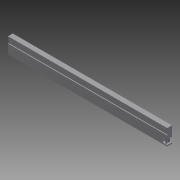
# Autodesk Inventor part: Bar
Saved by Autodesk Inventor 2012 (Build 160160000, 160)
## iProperties
Created: 2011-08-19
Part Number: Bar
Material: Default
Document SubType Name: Modeling
Designer: Minh Tran
Density: 1 g/cm^3
Author: Minh Tran
Autodesk Inventor part; units mm, degrees
ref_plane "YZ Plane" through (0, 0, 0) normal (1, 0, 0) x (0, 1, 0)
ref_plane "XZ Plane" through (0, 0, 0) normal (0, 1, 0) x (-1, 0, 0)
ref_plane "XY Plane" through (0, 0, 0) normal (0, 0, 1) x (1, 0, 0)
sketch "Sketch1" plane through (0, 0, 0) normal (0, 0, 1) x (1, 0, 0)
  line L0 (0, 0) -> (254, 0)
  line L1 (254, 0) -> (254, -25.4)
  line L2 (254, -25.4) -> (0, -25.4)
  line L3 (0, -25.4) -> (0, 0)
  dimension "d0" = 254
  dimension "d1" = 25.4
  constraints: 8 end point, 2 parallel, 1 horizontal, 1 perpendicular
  measures "d0" distance of L1.end L2.end
  measures "d1" distance of L0.end L1.end
extrude "Extrusion1" add sketch "Sketch1" along normal blind 7.62
sketch "Sketch2" plane through (0, 0, 7.62) normal (0, 0, 1) x (1, 0, 0)
  line L0 (0, -25.4) -> (0, 0) projected
  line L1 (0, -3.7895) -> (254, -3.7895)
  line L2 (254, -3.7895) -> (254, -10.1395)
  line L3 (254, -10.1395) -> (0, -10.1395)
  line L4 (0, -10.1395) -> (0, -3.7895)
  dimension "d4" = 254
  dimension "d5" = 6.35
  constraints: 8 end point, 2 parallel, 1 horizontal, 1 perpendicular, 1 point on line
  measures "d4" distance of L2.end L3.end
  measures "d5" distance of L1.end L2.end
extrude "Extrusion2" cut sketch "Sketch2" against normal blind 1.27
sketch "Sketch3" plane through (254, -25.4, 0) normal (1, 0, 0) x (0, 0, -1)
  line L0 (-7.62, 15.2605) -> (-7.62, 0) projected
  line L1 (-7.62, 2.0757) -> (0, 2.0757)
  line L2 (0, 2.0757) -> (0, 9.6957)
  line L3 (0, 9.6957) -> (-7.62, 9.6957)
  line L4 (-7.62, 9.6957) -> (-7.62, 2.0757)
  dimension "d8" = 7.62
  dimension "d9" = 7.62
  constraints: 8 end point, 2 parallel, 1 horizontal, 1 perpendicular, 1 point on line
  measures "d8" distance of L3.end L2.end
  measures "d9" distance of L2.end L1.end
extrude "Extrusion3" cut sketch "Sketch3" against normal blind 7.62
sketch "Sketch4" plane through (254, -23.3243, 7.62) normal (0, 1, 0) x (1, 0, 0)
  circle A0 centre (-3.2098, 1.884) radius 1.27
  circle A1 centre (-3.1463, 5.6104) radius 1.27
  point P0 (-254, 7.62)
  constraints: 2 centre point
extrude "Extrusion4" add sketch "Sketch4" along normal blind 7.62
body "Solid1"
